Autodesk Inventor part; units mm, degrees
(part 3 of 6)
  line L1773 (-14.7808, 26.7541) -> (-14.5927, 26.602)
  line L1774 (-14.5927, 26.602) -> (-14.4184, 26.455)
  line L1775 (-14.4184, 26.455) -> (-14.2558, 26.312)
  line L1776 (-14.2558, 26.312) -> (-14.1046, 26.1732)
  line L1777 (-14.1046, 26.1732) -> (-13.9666, 26.0412)
  line L1778 (-13.9666, 26.0412) -> (-13.8398, 25.9146)
  line L1779 (-13.8398, 25.9146) -> (-13.5974, 25.6603)
  line L1780 (-13.5974, 25.6603) -> (-13.5605, 25.6314)
  line L1781 (-13.5605, 25.6314) -> (-13.5287, 25.6153)
  line L1782 (-13.5287, 25.6153) -> (-13.5023, 25.6116)
  line L1783 (-13.5023, 25.6116) -> (-13.4865, 25.6168)
  line L1784 (-13.4865, 25.6168) -> (-13.143, 25.7946)
  line L1785 (-13.143, 25.7946) -> (-12.7973, 25.968)
  line L1786 (-12.7973, 25.968) -> (-12.7837, 25.9777)
  line L1787 (-12.7837, 25.9777) -> (-12.7712, 26.0012)
  line L1788 (-12.7712, 26.0012) -> (-12.7656, 26.0365)
  line L1789 (-12.7656, 26.0365) -> (-12.7672, 26.0833)
  line L1790 (-12.7672, 26.0833) -> (-12.8305, 26.4288)
  line L1791 (-12.8305, 26.4288) -> (-12.8584, 26.6059)
  line L1792 (-12.8584, 26.6059) -> (-12.8841, 26.7951)
  line L1793 (-12.8841, 26.7951) -> (-12.9075, 26.9989)
  line L1794 (-12.9075, 26.9989) -> (-12.9276, 27.2145)
  line L1795 (-12.9276, 27.2145) -> (-12.9441, 27.442)
  line L1796 (-12.9441, 27.442) -> (-12.9565, 27.6836)
  line L1797 (-12.9565, 27.6836) -> (-12.9642, 27.9367)
  line L1798 (-12.9642, 27.9367) -> (-12.9667, 28.1579)
  arc A57 (-12.249, 28.4774) -> (-12.9667, 28.1579) centre (0, 0) ccw
  line L1799 (-12.249, 28.4774) -> (-12.0862, 28.3276)
  line L1800 (-12.0862, 28.3276) -> (-11.9033, 28.1525)
  line L1801 (-11.9033, 28.1525) -> (-11.7321, 27.9817)
  line L1802 (-11.7321, 27.9817) -> (-11.5741, 27.8172)
  line L1803 (-11.5741, 27.8172) -> (-11.4273, 27.6579)
  line L1804 (-11.4273, 27.6579) -> (-11.2915, 27.5042)
  line L1805 (-11.2915, 27.5042) -> (-11.1681, 27.3584)
  line L1806 (-11.1681, 27.3584) -> (-11.0551, 27.2193)
  line L1807 (-11.0551, 27.2193) -> (-10.8407, 26.941)
  line L1808 (-10.8407, 26.941) -> (-10.807, 26.9085)
  line L1809 (-10.807, 26.9085) -> (-10.777, 26.8891)
  line L1810 (-10.777, 26.8891) -> (-10.7512, 26.8826)
  line L1811 (-10.7512, 26.8826) -> (-10.7349, 26.8862)
  line L1812 (-10.7349, 26.8862) -> (-10.3748, 27.0272)
  line L1813 (-10.3748, 27.0272) -> (-10.0128, 27.1634)
  line L1814 (-10.0128, 27.1634) -> (-9.9983, 27.1717)
  line L1815 (-9.9983, 27.1717) -> (-9.9834, 27.1937)
  line L1816 (-9.9834, 27.1937) -> (-9.9741, 27.2282)
  line L1817 (-9.9741, 27.2282) -> (-9.9708, 27.2749)
  line L1818 (-9.9708, 27.2749) -> (-9.9977, 27.6252)
  line L1819 (-9.9977, 27.6252) -> (-10.0069, 27.8042)
  line L1820 (-10.0069, 27.8042) -> (-10.0127, 27.995)
  line L1821 (-10.0127, 27.995) -> (-10.0146, 28.2002)
  line L1822 (-10.0146, 28.2002) -> (-10.0121, 28.4168)
  line L1823 (-10.0121, 28.4168) -> (-10.0047, 28.6447)
  line L1824 (-10.0047, 28.6447) -> (-9.9918, 28.8863)
  line L1825 (-9.9918, 28.8863) -> (-9.973, 29.1388)
  line L1826 (-9.973, 29.1388) -> (-9.9523, 29.359)
  arc A58 (-9.2052, 29.6018) -> (-9.9523, 29.359) centre (0, 0) ccw
  line L1827 (-9.2052, 29.6018) -> (-9.059, 29.4358)
  line L1828 (-9.059, 29.4358) -> (-8.8954, 29.2425)
  line L1829 (-8.8954, 29.2425) -> (-8.7429, 29.0547)
  line L1830 (-8.7429, 29.0547) -> (-8.603, 28.8746)
  line L1831 (-8.603, 28.8746) -> (-8.4737, 28.7009)
  line L1832 (-8.4737, 28.7009) -> (-8.3547, 28.5338)
  line L1833 (-8.3547, 28.5338) -> (-8.2472, 28.3759)
  line L1834 (-8.2472, 28.3759) -> (-8.1494, 28.2257)
  line L1835 (-8.1494, 28.2257) -> (-7.9652, 27.9266)
  line L1836 (-7.9652, 27.9266) -> (-7.9351, 27.8907)
  line L1837 (-7.9351, 27.8907) -> (-7.9073, 27.8683)
  line L1838 (-7.9073, 27.8683) -> (-7.8823, 27.8592)
  line L1839 (-7.8823, 27.8592) -> (-7.8657, 27.861)
  line L1840 (-7.8657, 27.861) -> (-7.4928, 27.9636)
  line L1841 (-7.4928, 27.9636) -> (-7.1186, 28.0612)
  line L1842 (-7.1186, 28.0612) -> (-7.1033, 28.0679)
  line L1843 (-7.1033, 28.0679) -> (-7.0862, 28.0883)
  line L1844 (-7.0862, 28.0883) -> (-7.0733, 28.1216)
  line L1845 (-7.0733, 28.1216) -> (-7.0652, 28.1677)
  line L1846 (-7.0652, 28.1677) -> (-7.0553, 28.5189)
  line L1847 (-7.0553, 28.5189) -> (-7.0457, 28.6979)
  line L1848 (-7.0457, 28.6979) -> (-7.0315, 28.8883)
  line L1849 (-7.0315, 28.8883) -> (-7.012, 29.0926)
  line L1850 (-7.012, 29.0926) -> (-6.9869, 29.3077)
  line L1851 (-6.9869, 29.3077) -> (-6.9557, 29.5336)
  line L1852 (-6.9557, 29.5336) -> (-6.9177, 29.7725)
  line L1853 (-6.9177, 29.7725) -> (-6.8726, 30.0216)
  line L1854 (-6.8726, 30.0216) -> (-6.829, 30.2385)
  arc A59 (-6.0605, 30.4018) -> (-6.829, 30.2385) centre (0, 0) ccw
  line L1855 (-6.0605, 30.4018) -> (-5.9325, 30.2214)
  line L1856 (-5.9325, 30.2214) -> (-5.79, 30.0122)
  line L1857 (-5.79, 30.0122) -> (-5.658, 29.8094)
  line L1858 (-5.658, 29.8094) -> (-5.5376, 29.6157)
  line L1859 (-5.5376, 29.6157) -> (-5.4272, 29.4294)
  line L1860 (-5.4272, 29.4294) -> (-5.3263, 29.2508)
  line L1861 (-5.3263, 29.2508) -> (-5.2359, 29.0826)
  line L1862 (-5.2359, 29.0826) -> (-5.1544, 28.9229)
  line L1863 (-5.1544, 28.9229) -> (-5.0025, 28.6062)
  line L1864 (-5.0025, 28.6062) -> (-4.9763, 28.5674)
  line L1865 (-4.9763, 28.5674) -> (-4.951, 28.5421)
  line L1866 (-4.951, 28.5421) -> (-4.927, 28.5305)
  line L1867 (-4.927, 28.5305) -> (-4.9104, 28.5306)
  line L1868 (-4.9104, 28.5306) -> (-4.5288, 28.5936)
  line L1869 (-4.5288, 28.5936) -> (-4.1464, 28.6516)
  line L1870 (-4.1464, 28.6516) -> (-4.1305, 28.6567)
  line L1871 (-4.1305, 28.6567) -> (-4.1114, 28.6751)
  line L1872 (-4.1114, 28.6751) -> (-4.0951, 28.7069)
  line L1873 (-4.0951, 28.7069) -> (-4.0822, 28.7519)
  line L1874 (-4.0822, 28.7519) -> (-4.0356, 29.1001)
  line L1875 (-4.0356, 29.1001) -> (-4.0074, 29.2771)
  line L1876 (-4.0074, 29.2771) -> (-3.9734, 29.465)
  line L1877 (-3.9734, 29.465) -> (-3.9326, 29.6661)
  line L1878 (-3.9326, 29.6661) -> (-3.8852, 29.8774)
  line L1879 (-3.8852, 29.8774) -> (-3.8305, 30.0989)
  line L1880 (-3.8305, 30.0989) -> (-3.7677, 30.3325)
  line L1881 (-3.7677, 30.3325) -> (-3.6968, 30.5755)
  line L1882 (-3.6968, 30.5755) -> (-3.6308, 30.7866)
  arc A60 (-2.8495, 30.8688) -> (-3.6308, 30.7866) centre (0, 0) ccw
  line L1883 (-2.8495, 30.8688) -> (-2.741, 30.676)
  line L1884 (-2.741, 30.676) -> (-2.6211, 30.453)
  line L1885 (-2.6211, 30.453) -> (-2.5111, 30.2376)
  line L1886 (-2.5111, 30.2376) -> (-2.4116, 30.0323)
  line L1887 (-2.4116, 30.0323) -> (-2.3213, 29.8355)
  line L1888 (-2.3213, 29.8355) -> (-2.2396, 29.6473)
  line L1889 (-2.2396, 29.6473) -> (-2.1673, 29.4705)
  line L1890 (-2.1673, 29.4705) -> (-2.1029, 29.3033)
  line L1891 (-2.1029, 29.3033) -> (-1.9849, 28.9724)
  line L1892 (-1.9849, 28.9724) -> (-1.9629, 28.931)
  line L1893 (-1.9629, 28.931) -> (-1.9404, 28.9033)
  line L1894 (-1.9404, 28.9033) -> (-1.9178, 28.8892)
  line L1895 (-1.9178, 28.8892) -> (-1.9012, 28.8876)
  line L1896 (-1.9012, 28.8876) -> (-1.5151, 28.9103)
  line L1897 (-1.5151, 28.9103) -> (-1.1288, 28.9281)
  line L1898 (-1.1288, 28.9281) -> (-1.1124, 28.9314)
  line L1899 (-1.1124, 28.9314) -> (-1.0915, 28.9478)
  line L1900 (-1.0915, 28.9478) -> (-1.0719, 28.9777)
  line L1901 (-1.0719, 28.9777) -> (-1.0544, 29.0211)
  line L1902 (-1.0544, 29.0211) -> (-0.9717, 29.3626)
  line L1903 (-0.9717, 29.3626) -> (-0.9251, 29.5356)
  line L1904 (-0.9251, 29.5356) -> (-0.8717, 29.719)
  line L1905 (-0.8717, 29.719) -> (-0.8101, 29.9147)
  line L1906 (-0.8101, 29.9147) -> (-0.7408, 30.1199)
  line L1907 (-0.7408, 30.1199) -> (-0.6634, 30.3344)
  line L1908 (-0.6634, 30.3344) -> (-0.5765, 30.5601)
  line L1909 (-0.5765, 30.5601) -> (-0.4805, 30.7945)
  line L1910 (-0.4805, 30.7945) -> (-0.3928, 30.9975)
  arc A61 (0.3928, 30.9975) -> (-0.3928, 30.9975) centre (0, 0) ccw
  line L1911 (0.3928, 30.9975) -> (0.4805, 30.7945)
  line L1912 (0.4805, 30.7945) -> (0.5765, 30.5601)
  line L1913 (0.5765, 30.5601) -> (0.6634, 30.3344)
  line L1914 (0.6634, 30.3344) -> (0.7408, 30.1199)
  line L1915 (0.7408, 30.1199) -> (0.8101, 29.9147)
  line L1916 (0.8101, 29.9147) -> (0.8717, 29.719)
  line L1917 (0.8717, 29.719) -> (0.9251, 29.5356)
  line L1918 (0.9251, 29.5356) -> (0.9717, 29.3626)
  line L1919 (0.9717, 29.3626) -> (1.0544, 29.0211)
  line L1920 (1.0544, 29.0211) -> (1.0719, 28.9777)
  line L1921 (1.0719, 28.9777) -> (1.0915, 28.9478)
  line L1922 (1.0915, 28.9478) -> (1.1124, 28.9314)
  line L1923 (1.1124, 28.9314) -> (1.1288, 28.9281)
  line L1924 (1.1288, 28.9281) -> (1.5151, 28.9103)
  line L1925 (1.5151, 28.9103) -> (1.9012, 28.8876)
  line L1926 (1.9012, 28.8876) -> (1.9178, 28.8892)
  line L1927 (1.9178, 28.8892) -> (1.9404, 28.9033)
  line L1928 (1.9404, 28.9033) -> (1.9629, 28.931)
  line L1929 (1.9629, 28.931) -> (1.9849, 28.9724)
  line L1930 (1.9849, 28.9724) -> (2.1029, 29.3033)
  line L1931 (2.1029, 29.3033) -> (2.1673, 29.4705)
  line L1932 (2.1673, 29.4705) -> (2.2396, 29.6473)
  line L1933 (2.2396, 29.6473) -> (2.3213, 29.8355)
  line L1934 (2.3213, 29.8355) -> (2.4116, 30.0323)
  line L1935 (2.4116, 30.0323) -> (2.5111, 30.2376)
  line L1936 (2.5111, 30.2376) -> (2.6211, 30.453)
  line L1937 (2.6211, 30.453) -> (2.741, 30.676)
  line L1938 (2.741, 30.676) -> (2.8495, 30.8688)
  arc A62 (3.6308, 30.7866) -> (2.8495, 30.8688) centre (0, 0) ccw
  line L1939 (3.6308, 30.7866) -> (3.6968, 30.5755)
  line L1940 (3.6968, 30.5755) -> (3.7677, 30.3325)
  line L1941 (3.7677, 30.3325) -> (3.8305, 30.0989)
  line L1942 (3.8305, 30.0989) -> (3.8852, 29.8774)
  line L1943 (3.8852, 29.8774) -> (3.9326, 29.6661)
  line L1944 (3.9326, 29.6661) -> (3.9734, 29.465)
  line L1945 (3.9734, 29.465) -> (4.0074, 29.2771)
  line L1946 (4.0074, 29.2771) -> (4.0356, 29.1001)
  line L1947 (4.0356, 29.1001) -> (4.0822, 28.7519)
  line L1948 (4.0822, 28.7519) -> (4.0951, 28.7069)
  line L1949 (4.0951, 28.7069) -> (4.1114, 28.6751)
  line L1950 (4.1114, 28.6751) -> (4.1305, 28.6567)
  line L1951 (4.1305, 28.6567) -> (4.1464, 28.6516)
  line L1952 (4.1464, 28.6516) -> (4.5288, 28.5936)
  line L1953 (4.5288, 28.5936) -> (4.9104, 28.5306)
  line L1954 (4.9104, 28.5306) -> (4.927, 28.5305)
  line L1955 (4.927, 28.5305) -> (4.951, 28.5421)
  line L1956 (4.951, 28.5421) -> (4.9763, 28.5674)
  line L1957 (4.9763, 28.5674) -> (5.0025, 28.6062)
  line L1958 (5.0025, 28.6062) -> (5.1544, 28.9229)
  line L1959 (5.1544, 28.9229) -> (5.2359, 29.0826)
  line L1960 (5.2359, 29.0826) -> (5.3263, 29.2508)
  line L1961 (5.3263, 29.2508) -> (5.4272, 29.4294)
  line L1962 (5.4272, 29.4294) -> (5.5376, 29.6157)
  line L1963 (5.5376, 29.6157) -> (5.658, 29.8094)
  line L1964 (5.658, 29.8094) -> (5.79, 30.0122)
  line L1965 (5.79, 30.0122) -> (5.9325, 30.2214)
  line L1966 (5.9325, 30.2214) -> (6.0605, 30.4018)
  arc A63 (6.829, 30.2385) -> (6.0605, 30.4018) centre (0, 0) ccw
  line L1967 (6.829, 30.2385) -> (6.8726, 30.0216)
  line L1968 (6.8726, 30.0216) -> (6.9177, 29.7725)
  line L1969 (6.9177, 29.7725) -> (6.9557, 29.5336)
  line L1970 (6.9557, 29.5336) -> (6.9869, 29.3077)
  line L1971 (6.9869, 29.3077) -> (7.012, 29.0926)
  line L1972 (7.012, 29.0926) -> (7.0315, 28.8883)
  line L1973 (7.0315, 28.8883) -> (7.0457, 28.6979)
  line L1974 (7.0457, 28.6979) -> (7.0553, 28.5189)
  line L1975 (7.0553, 28.5189) -> (7.0652, 28.1677)
  line L1976 (7.0652, 28.1677) -> (7.0733, 28.1216)
  line L1977 (7.0733, 28.1216) -> (7.0862, 28.0883)
  line L1978 (7.0862, 28.0883) -> (7.1033, 28.0679)
  line L1979 (7.1033, 28.0679) -> (7.1186, 28.0612)
  line L1980 (7.1186, 28.0612) -> (7.4928, 27.9636)
  line L1981 (7.4928, 27.9636) -> (7.8657, 27.861)
  line L1982 (7.8657, 27.861) -> (7.8823, 27.8592)
  line L1983 (7.8823, 27.8592) -> (7.9073, 27.8683)
  line L1984 (7.9073, 27.8683) -> (7.9351, 27.8907)
  line L1985 (7.9351, 27.8907) -> (7.9652, 27.9266)
  line L1986 (7.9652, 27.9266) -> (8.1494, 28.2257)
  line L1987 (8.1494, 28.2257) -> (8.2472, 28.3759)
  line L1988 (8.2472, 28.3759) -> (8.3547, 28.5338)
  line L1989 (8.3547, 28.5338) -> (8.4737, 28.7009)
  line L1990 (8.4737, 28.7009) -> (8.603, 28.8746)
  line L1991 (8.603, 28.8746) -> (8.7429, 29.0547)
  line L1992 (8.7429, 29.0547) -> (8.8954, 29.2425)
  line L1993 (8.8954, 29.2425) -> (9.059, 29.4358)
  line L1994 (9.059, 29.4358) -> (9.2052, 29.6018)
  arc A64 (9.9523, 29.359) -> (9.2052, 29.6018) centre (0, 0) ccw
  line L1995 (9.9523, 29.359) -> (9.973, 29.1388)
  line L1996 (9.973, 29.1388) -> (9.9918, 28.8863)
  line L1997 (9.9918, 28.8863) -> (10.0047, 28.6447)
  line L1998 (10.0047, 28.6447) -> (10.0121, 28.4168)
  line L1999 (10.0121, 28.4168) -> (10.0146, 28.2002)
  line L2000 (10.0146, 28.2002) -> (10.0127, 27.995)
  line L2001 (10.0127, 27.995) -> (10.0069, 27.8042)
  line L2002 (10.0069, 27.8042) -> (9.9977, 27.6252)
  line L2003 (9.9977, 27.6252) -> (9.9708, 27.2749)
  line L2004 (9.9708, 27.2749) -> (9.9741, 27.2282)
  line L2005 (9.9741, 27.2282) -> (9.9834, 27.1937)
  line L2006 (9.9834, 27.1937) -> (9.9983, 27.1717)
  line L2007 (9.9983, 27.1717) -> (10.0128, 27.1634)
  line L2008 (10.0128, 27.1634) -> (10.3748, 27.0272)
  line L2009 (10.3748, 27.0272) -> (10.7349, 26.8862)
  line L2010 (10.7349, 26.8862) -> (10.7512, 26.8826)
  line L2011 (10.7512, 26.8826) -> (10.777, 26.8891)
  line L2012 (10.777, 26.8891) -> (10.807, 26.9085)
  line L2013 (10.807, 26.9085) -> (10.8407, 26.941)
  line L2014 (10.8407, 26.941) -> (11.0551, 27.2193)
  line L2015 (11.0551, 27.2193) -> (11.1681, 27.3584)
  line L2016 (11.1681, 27.3584) -> (11.2915, 27.5042)
  line L2017 (11.2915, 27.5042) -> (11.4273, 27.6579)
  line L2018 (11.4273, 27.6579) -> (11.5741, 27.8172)
  line L2019 (11.5741, 27.8172) -> (11.7321, 27.9817)
  line L2020 (11.7321, 27.9817) -> (11.9033, 28.1525)
  line L2021 (11.9033, 28.1525) -> (12.0862, 28.3276)
  line L2022 (12.0862, 28.3276) -> (12.249, 28.4774)
  arc A65 (12.9667, 28.1579) -> (12.249, 28.4774) centre (0, 0) ccw
  line L2023 (12.9667, 28.1579) -> (12.9642, 27.9367)
  line L2024 (12.9642, 27.9367) -> (12.9565, 27.6836)
  line L2025 (12.9565, 27.6836) -> (12.9441, 27.442)
  line L2026 (12.9441, 27.442) -> (12.9276, 27.2145)
  line L2027 (12.9276, 27.2145) -> (12.9075, 26.9989)
  line L2028 (12.9075, 26.9989) -> (12.8841, 26.7951)
  line L2029 (12.8841, 26.7951) -> (12.8584, 26.6059)
  line L2030 (12.8584, 26.6059) -> (12.8305, 26.4288)
  line L2031 (12.8305, 26.4288) -> (12.7672, 26.0833)
  line L2032 (12.7672, 26.0833) -> (12.7656, 26.0365)
  line L2033 (12.7656, 26.0365) -> (12.7712, 26.0012)
  line L2034 (12.7712, 26.0012) -> (12.7837, 25.9777)
  line L2035 (12.7837, 25.9777) -> (12.7973, 25.968)
  line L2036 (12.7973, 25.968) -> (13.143, 25.7946)
  line L2037 (13.143, 25.7946) -> (13.4865, 25.6168)
  line L2038 (13.4865, 25.6168) -> (13.5023, 25.6116)
  line L2039 (13.5023, 25.6116) -> (13.5287, 25.6153)
  line L2040 (13.5287, 25.6153) -> (13.5605, 25.6314)
  line L2041 (13.5605, 25.6314) -> (13.5974, 25.6603)
  line L2042 (13.5974, 25.6603) -> (13.8398, 25.9146)
  line L2043 (13.8398, 25.9146) -> (13.9666, 26.0412)
  line L2044 (13.9666, 26.0412) -> (14.1046, 26.1732)
  line L2045 (14.1046, 26.1732) -> (14.2558, 26.312)
  line L2046 (14.2558, 26.312) -> (14.4184, 26.455)
  line L2047 (14.4184, 26.455) -> (14.5927, 26.602)
  line L2048 (14.5927, 26.602) -> (14.7808, 26.7541)
  line L2049 (14.7808, 26.7541) -> (14.9811, 26.9091)
  line L2050 (14.9811, 26.9091) -> (15.1586, 27.041)
  arc A66 (15.8389, 26.6482) -> (15.1586, 27.041) centre (0, 0) ccw
  line L2051 (15.8389, 26.6482) -> (15.8134, 26.4285)
  line L2052 (15.8134, 26.4285) -> (15.7793, 26.1776)
  line L2053 (15.7793, 26.1776) -> (15.7417, 25.9387)
  line L2054 (15.7417, 25.9387) -> (15.7015, 25.7142)
  line L2055 (15.7015, 25.7142) -> (15.6589, 25.5018)
  line L2056 (15.6589, 25.5018) -> (15.6144, 25.3015)
  line L2057 (15.6144, 25.3015) -> (15.569, 25.1161)
  line L2058 (15.569, 25.1161) -> (15.5228, 24.9429)
  line L2059 (15.5228, 24.9429) -> (15.4237, 24.6058)
  line L2060 (15.4237, 24.6058) -> (15.4172, 24.5595)
  line L2061 (15.4172, 24.5595) -> (15.4191, 24.5238)
  line L2062 (15.4191, 24.5238) -> (15.4291, 24.4991)
  line L2063 (15.4291, 24.4991) -> (15.4416, 24.488)
  line L2064 (15.4416, 24.488) -> (15.7673, 24.2795)
  line L2065 (15.7673, 24.2795) -> (16.0903, 24.0668)
  line L2066 (16.0903, 24.0668) -> (16.1055, 24.0599)
  line L2067 (16.1055, 24.0599) -> (16.1321, 24.0608)
  line L2068 (16.1321, 24.0608) -> (16.1655, 24.0735)
  line L2069 (16.1655, 24.0735) -> (16.2052, 24.0984)
  line L2070 (16.2052, 24.0984) -> (16.4728, 24.326)
  line L2071 (16.4728, 24.326) -> (16.6122, 24.4386)
  line L2072 (16.6122, 24.4386) -> (16.7632, 24.5555)
  line L2073 (16.7632, 24.5555) -> (16.928, 24.6777)
  line L2074 (16.928, 24.6777) -> (17.1047, 24.8029)
  line L2075 (17.1047, 24.8029) -> (17.2934, 24.931)
  line L2076 (17.2934, 24.931) -> (17.4964, 25.0625)
  line L2077 (17.4964, 25.0625) -> (17.7118, 25.1957)
  line L2078 (17.7118, 25.1957) -> (17.9021, 25.3084)
  arc A67 (18.5377, 24.8466) -> (17.9021, 25.3084) centre (0, 0) ccw
  line L2079 (18.5377, 24.8466) -> (18.4893, 24.6308)
  line L2080 (18.4893, 24.6308) -> (18.4292, 24.3848)
  line L2081 (18.4292, 24.3848) -> (18.3668, 24.1511)
  line L2082 (18.3668, 24.1511) -> (18.3034, 23.932)
  line L2083 (18.3034, 23.932) -> (18.2388, 23.7253)
  line L2084 (18.2388, 23.7253) -> (18.1736, 23.5308)
  line L2085 (18.1736, 23.5308) -> (18.1091, 23.3511)
  line L2086 (18.1091, 23.3511) -> (18.045, 23.1837)
  line L2087 (18.045, 23.1837) -> (17.9112, 22.8588)
  line L2088 (17.9112, 22.8588) -> (17.8999, 22.8134)
  line L2089 (17.8999, 22.8134) -> (17.8981, 22.7777)
  line L2090 (17.8981, 22.7777) -> (17.9055, 22.7521)
  line L2091 (17.9055, 22.7521) -> (17.9167, 22.7398)
  line L2092 (17.9167, 22.7398) -> (18.2188, 22.4984)
  line L2093 (18.2188, 22.4984) -> (18.5178, 22.2531)
  line L2094 (18.5178, 22.2531) -> (18.5322, 22.2446)
  line L2095 (18.5322, 22.2446) -> (18.5587, 22.2427)
  line L2096 (18.5587, 22.2427) -> (18.5933, 22.2519)
  line L2097 (18.5933, 22.2519) -> (18.6353, 22.2724)
  line L2098 (18.6353, 22.2724) -> (18.9253, 22.4708)
  line L2099 (18.9253, 22.4708) -> (19.0757, 22.5683)
  line L2100 (19.0757, 22.5683) -> (19.2381, 22.6688)
  line L2101 (19.2381, 22.6688) -> (19.4148, 22.773)
  line L2102 (19.4148, 22.773) -> (19.6036, 22.8791)
  line L2103 (19.6036, 22.8791) -> (19.8047, 22.9867)
  line L2104 (19.8047, 22.9867) -> (20.0203, 23.0963)
  line L2105 (20.0203, 23.0963) -> (20.2484, 23.2063)
  line L2106 (20.2484, 23.2063) -> (20.4495, 23.2985)
  arc A68 (21.0333, 22.7728) -> (20.4495, 23.2985) centre (0, 0) ccw
  line L2107 (21.0333, 22.7728) -> (20.9626, 22.5632)
  line L2108 (20.9626, 22.5632) -> (20.8771, 22.3249)
  line L2109 (20.8771, 22.3249) -> (20.7906, 22.099)
  line L2110 (20.7906, 22.099) -> (20.7047, 21.8877)
  line L2111 (20.7047, 21.8877) -> (20.6189, 21.6889)
  line L2112 (20.6189, 21.6889) -> (20.5336, 21.5022)
  line L2113 (20.5336, 21.5022) -> (20.4507, 21.3302)
  line L2114 (20.4507, 21.3302) -> (20.3695, 21.1705)
  line L2115 (20.3695, 21.1705) -> (20.2025, 20.8614)
  line L2116 (20.2025, 20.8614) -> (20.1865, 20.8174)
  line L2117 (20.1865, 20.8174) -> (20.181, 20.7821)
  line L2118 (20.181, 20.7821) -> (20.1856, 20.7559)
  line L2119 (20.1856, 20.7559) -> (20.1955, 20.7424)
  line L2120 (20.1955, 20.7424) -> (20.4707, 20.4707)
  line L2121 (20.4707, 20.4707) -> (20.7424, 20.1955)
  line L2122 (20.7424, 20.1955) -> (20.7559, 20.1856)
  line L2123 (20.7559, 20.1856) -> (20.7821, 20.181)
  line L2124 (20.7821, 20.181) -> (20.8174, 20.1865)
  line L2125 (20.8174, 20.1865) -> (20.8614, 20.2025)
  line L2126 (20.8614, 20.2025) -> (21.1705, 20.3695)
  line L2127 (21.1705, 20.3695) -> (21.3302, 20.4507)
  line L2128 (21.3302, 20.4507) -> (21.5022, 20.5336)
  line L2129 (21.5022, 20.5336) -> (21.6889, 20.6189)
  line L2130 (21.6889, 20.6189) -> (21.8877, 20.7047)
  line L2131 (21.8877, 20.7047) -> (22.099, 20.7906)
  line L2132 (22.099, 20.7906) -> (22.3249, 20.8771)
  line L2133 (22.3249, 20.8771) -> (22.5632, 20.9626)
  line L2134 (22.5632, 20.9626) -> (22.7728, 21.0333)
  arc A69 (23.2985, 20.4495) -> (22.7728, 21.0333) centre (0, 0) ccw
  line L2135 (23.2985, 20.4495) -> (23.2063, 20.2484)
  line L2136 (23.2063, 20.2484) -> (23.0963, 20.0203)
  line L2137 (23.0963, 20.0203) -> (22.9867, 19.8047)
  line L2138 (22.9867, 19.8047) -> (22.8791, 19.6036)
  line L2139 (22.8791, 19.6036) -> (22.773, 19.4148)
  line L2140 (22.773, 19.4148) -> (22.6688, 19.2381)
  line L2141 (22.6688, 19.2381) -> (22.5683, 19.0757)
  line L2142 (22.5683, 19.0757) -> (22.4708, 18.9253)
  line L2143 (22.4708, 18.9253) -> (22.2724, 18.6353)
  line L2144 (22.2724, 18.6353) -> (22.2519, 18.5933)
  line L2145 (22.2519, 18.5933) -> (22.2427, 18.5587)
  line L2146 (22.2427, 18.5587) -> (22.2446, 18.5322)
  line L2147 (22.2446, 18.5322) -> (22.2531, 18.5178)
  line L2148 (22.2531, 18.5178) -> (22.4984, 18.2188)
  line L2149 (22.4984, 18.2188) -> (22.7398, 17.9167)
  line L2150 (22.7398, 17.9167) -> (22.7521, 17.9055)
  line L2151 (22.7521, 17.9055) -> (22.7777, 17.8981)
  line L2152 (22.7777, 17.8981) -> (22.8134, 17.8999)
  line L2153 (22.8134, 17.8999) -> (22.8588, 17.9112)
  line L2154 (22.8588, 17.9112) -> (23.1837, 18.045)
  line L2155 (23.1837, 18.045) -> (23.3511, 18.1091)
  line L2156 (23.3511, 18.1091) -> (23.5308, 18.1736)
  line L2157 (23.5308, 18.1736) -> (23.7253, 18.2388)
  line L2158 (23.7253, 18.2388) -> (23.932, 18.3034)
  line L2159 (23.932, 18.3034) -> (24.1511, 18.3668)
  line L2160 (24.1511, 18.3668) -> (24.3848, 18.4292)
  line L2161 (24.3848, 18.4292) -> (24.6308, 18.4893)
  line L2162 (24.6308, 18.4893) -> (24.8466, 18.5377)
  arc A70 (25.3084, 17.9021) -> (24.8466, 18.5377) centre (0, 0) ccw
  line L2163 (25.3084, 17.9021) -> (25.1957, 17.7118)
  line L2164 (25.1957, 17.7118) -> (25.0625, 17.4964)
  line L2165 (25.0625, 17.4964) -> (24.931, 17.2934)
  line L2166 (24.931, 17.2934) -> (24.8029, 17.1047)
  line L2167 (24.8029, 17.1047) -> (24.6777, 16.928)
  line L2168 (24.6777, 16.928) -> (24.5555, 16.7632)
  line L2169 (24.5555, 16.7632) -> (24.4386, 16.6122)
  line L2170 (24.4386, 16.6122) -> (24.326, 16.4728)
  line L2171 (24.326, 16.4728) -> (24.0984, 16.2052)
  line L2172 (24.0984, 16.2052) -> (24.0735, 16.1655)
  line L2173 (24.0735, 16.1655) -> (24.0608, 16.1321)
  line L2174 (24.0608, 16.1321) -> (24.0599, 16.1055)
  line L2175 (24.0599, 16.1055) -> (24.0668, 16.0903)
  line L2176 (24.0668, 16.0903) -> (24.2795, 15.7673)
  line L2177 (24.2795, 15.7673) -> (24.488, 15.4416)
  line L2178 (24.488, 15.4416) -> (24.4991, 15.4291)
  line L2179 (24.4991, 15.4291) -> (24.5238, 15.4191)
  line L2180 (24.5238, 15.4191) -> (24.5595, 15.4172)
  line L2181 (24.5595, 15.4172) -> (24.6058, 15.4237)
  line L2182 (24.6058, 15.4237) -> (24.9429, 15.5228)
  line L2183 (24.9429, 15.5228) -> (25.1161, 15.569)
  line L2184 (25.1161, 15.569) -> (25.3015, 15.6144)
  line L2185 (25.3015, 15.6144) -> (25.5018, 15.6589)
  line L2186 (25.5018, 15.6589) -> (25.7142, 15.7015)
  line L2187 (25.7142, 15.7015) -> (25.9387, 15.7417)
  line L2188 (25.9387, 15.7417) -> (26.1776, 15.7793)
  line L2189 (26.1776, 15.7793) -> (26.4285, 15.8134)
  line L2190 (26.4285, 15.8134) -> (26.6482, 15.8389)
  arc A71 (27.041, 15.1586) -> (26.6482, 15.8389) centre (0, 0) ccw
  line L2191 (27.041, 15.1586) -> (26.9091, 14.9811)
  line L2192 (26.9091, 14.9811) -> (26.7541, 14.7808)
  line L2193 (26.7541, 14.7808) -> (26.602, 14.5927)
  line L2194 (26.602, 14.5927) -> (26.455, 14.4184)
  line L2195 (26.455, 14.4184) -> (26.312, 14.2558)
  line L2196 (26.312, 14.2558) -> (26.1732, 14.1046)
  line L2197 (26.1732, 14.1046) -> (26.0412, 13.9666)
  line L2198 (26.0412, 13.9666) -> (25.9146, 13.8398)
  line L2199 (25.9146, 13.8398) -> (25.6603, 13.5974)
  line L2200 (25.6603, 13.5974) -> (25.6314, 13.5605)
  line L2201 (25.6314, 13.5605) -> (25.6153, 13.5287)
  line L2202 (25.6153, 13.5287) -> (25.6116, 13.5023)
  line L2203 (25.6116, 13.5023) -> (25.6168, 13.4865)
  line L2204 (25.6168, 13.4865) -> (25.7946, 13.143)
  line L2205 (25.7946, 13.143) -> (25.968, 12.7973)
  line L2206 (25.968, 12.7973) -> (25.9777, 12.7837)
  line L2207 (25.9777, 12.7837) -> (26.0012, 12.7712)
  line L2208 (26.0012, 12.7712) -> (26.0365, 12.7656)
  line L2209 (26.0365, 12.7656) -> (26.0833, 12.7672)
  line L2210 (26.0833, 12.7672) -> (26.4288, 12.8305)
  line L2211 (26.4288, 12.8305) -> (26.6059, 12.8584)
  line L2212 (26.6059, 12.8584) -> (26.7951, 12.8841)
  line L2213 (26.7951, 12.8841) -> (26.9989, 12.9075)
  line L2214 (26.9989, 12.9075) -> (27.2145, 12.9276)
  line L2215 (27.2145, 12.9276) -> (27.442, 12.9441)
  line L2216 (27.442, 12.9441) -> (27.6836, 12.9565)
  line L2217 (27.6836, 12.9565) -> (27.9367, 12.9642)
  line L2218 (27.9367, 12.9642) -> (28.1579, 12.9667)
  arc A72 (28.4774, 12.249) -> (28.1579, 12.9667) centre (0, 0) ccw
  line L2219 (28.4774, 12.249) -> (28.3276, 12.0862)
  line L2220 (28.3276, 12.0862) -> (28.1525, 11.9033)
  line L2221 (28.1525, 11.9033) -> (27.9817, 11.7321)
  line L2222 (27.9817, 11.7321) -> (27.8172, 11.5741)
  line L2223 (27.8172, 11.5741) -> (27.6579, 11.4273)
  line L2224 (27.6579, 11.4273) -> (27.5042, 11.2915)
  line L2225 (27.5042, 11.2915) -> (27.3584, 11.1681)
  line L2226 (27.3584, 11.1681) -> (27.2193, 11.0551)
  line L2227 (27.2193, 11.0551) -> (26.941, 10.8407)
  line L2228 (26.941, 10.8407) -> (26.9085, 10.807)
  line L2229 (26.9085, 10.807) -> (26.8891, 10.777)
  line L2230 (26.8891, 10.777) -> (26.8826, 10.7512)
  line L2231 (26.8826, 10.7512) -> (26.8862, 10.7349)
  line L2232 (26.8862, 10.7349) -> (27.0272, 10.3748)
  line L2233 (27.0272, 10.3748) -> (27.1634, 10.0128)
  line L2234 (27.1634, 10.0128) -> (27.1717, 9.9983)
  line L2235 (27.1717, 9.9983) -> (27.1937, 9.9834)
  line L2236 (27.1937, 9.9834) -> (27.2282, 9.9741)
  line L2237 (27.2282, 9.9741) -> (27.2749, 9.9708)
  line L2238 (27.2749, 9.9708) -> (27.6252, 9.9977)
  line L2239 (27.6252, 9.9977) -> (27.8042, 10.0069)
  line L2240 (27.8042, 10.0069) -> (27.995, 10.0127)
  line L2241 (27.995, 10.0127) -> (28.2002, 10.0146)
  line L2242 (28.2002, 10.0146) -> (28.4168, 10.0121)
  line L2243 (28.4168, 10.0121) -> (28.6447, 10.0047)
  line L2244 (28.6447, 10.0047) -> (28.8863, 9.9918)
  line L2245 (28.8863, 9.9918) -> (29.1388, 9.973)
  line L2246 (29.1388, 9.973) -> (29.359, 9.9523)
  arc A73 (29.6018, 9.2052) -> (29.359, 9.9523) centre (0, 0) ccw
  line L2247 (29.6018, 9.2052) -> (29.4358, 9.059)
  line L2248 (29.4358, 9.059) -> (29.2425, 8.8954)
  line L2249 (29.2425, 8.8954) -> (29.0547, 8.7429)
  line L2250 (29.0547, 8.7429) -> (28.8746, 8.603)
  line L2251 (28.8746, 8.603) -> (28.7009, 8.4737)
  line L2252 (28.7009, 8.4737) -> (28.5338, 8.3547)
  line L2253 (28.5338, 8.3547) -> (28.3759, 8.2472)
  line L2254 (28.3759, 8.2472) -> (28.2257, 8.1494)
  line L2255 (28.2257, 8.1494) -> (27.9266, 7.9652)
  line L2256 (27.9266, 7.9652) -> (27.8907, 7.9351)
  line L2257 (27.8907, 7.9351) -> (27.8683, 7.9073)
  line L2258 (27.8683, 7.9073) -> (27.8592, 7.8823)
  line L2259 (27.8592, 7.8823) -> (27.861, 7.8657)
  line L2260 (27.861, 7.8657) -> (27.9636, 7.4928)
  line L2261 (27.9636, 7.4928) -> (28.0612, 7.1186)
  line L2262 (28.0612, 7.1186) -> (28.0679, 7.1033)
  line L2263 (28.0679, 7.1033) -> (28.0883, 7.0862)
  line L2264 (28.0883, 7.0862) -> (28.1216, 7.0733)
  line L2265 (28.1216, 7.0733) -> (28.1677, 7.0652)
  line L2266 (28.1677, 7.0652) -> (28.5189, 7.0553)
  line L2267 (28.5189, 7.0553) -> (28.6979, 7.0457)
  line L2268 (28.6979, 7.0457) -> (28.8883, 7.0315)
  line L2269 (28.8883, 7.0315) -> (29.0926, 7.012)
  line L2270 (29.0926, 7.012) -> (29.3077, 6.9869)
  line L2271 (29.3077, 6.9869) -> (29.5336, 6.9557)
  line L2272 (29.5336, 6.9557) -> (29.7725, 6.9177)
  line L2273 (29.7725, 6.9177) -> (30.0216, 6.8726)
  line L2274 (30.0216, 6.8726) -> (30.2385, 6.829)
  arc A74 (30.4018, 6.0605) -> (30.2385, 6.829) centre (0, 0) ccw
  line L2275 (30.4018, 6.0605) -> (30.2214, 5.9325)
  line L2276 (30.2214, 5.9325) -> (30.0122, 5.79)
  line L2277 (30.0122, 5.79) -> (29.8094, 5.658)
  line L2278 (29.8094, 5.658) -> (29.6157, 5.5376)
  line L2279 (29.6157, 5.5376) -> (29.4294, 5.4272)
  line L2280 (29.4294, 5.4272) -> (29.2508, 5.3263)
  line L2281 (29.2508, 5.3263) -> (29.0826, 5.2359)
  line L2282 (29.0826, 5.2359) -> (28.9229, 5.1544)
  line L2283 (28.9229, 5.1544) -> (28.6062, 5.0025)
  line L2284 (28.6062, 5.0025) -> (28.5674, 4.9763)
  line L2285 (28.5674, 4.9763) -> (28.5421, 4.951)
  line L2286 (28.5421, 4.951) -> (28.5305, 4.927)
  line L2287 (28.5305, 4.927) -> (28.5306, 4.9104)
  line L2288 (28.5306, 4.9104) -> (28.5936, 4.5288)
  line L2289 (28.5936, 4.5288) -> (28.6516, 4.1464)
  line L2290 (28.6516, 4.1464) -> (28.6567, 4.1305)
  line L2291 (28.6567, 4.1305) -> (28.6751, 4.1114)
  line L2292 (28.6751, 4.1114) -> (28.7069, 4.0951)
  line L2293 (28.7069, 4.0951) -> (28.7519, 4.0822)
  line L2294 (28.7519, 4.0822) -> (29.1001, 4.0356)
  line L2295 (29.1001, 4.0356) -> (29.2771, 4.0074)
  line L2296 (29.2771, 4.0074) -> (29.465, 3.9734)
  line L2297 (29.465, 3.9734) -> (29.6661, 3.9326)
  line L2298 (29.6661, 3.9326) -> (29.8774, 3.8852)
  line L2299 (29.8774, 3.8852) -> (30.0989, 3.8305)
  line L2300 (30.0989, 3.8305) -> (30.3325, 3.7677)
  line L2301 (30.3325, 3.7677) -> (30.5755, 3.6968)
  line L2302 (30.5755, 3.6968) -> (30.7866, 3.6308)
  arc A75 (30.8688, 2.8495) -> (30.7866, 3.6308) centre (0, 0) ccw
  line L2303 (30.8688, 2.8495) -> (30.676, 2.741)
  line L2304 (30.8694, -4.5708) -> (30.9098, -4.4161)
  line L2305 (30.9098, -4.4161) -> (30.9538, -4.2725)
  line L2306 (30.9538, -4.2725) -> (31.0003, -4.1408)
  line L2307 (31.0003, -4.1408) -> (31.0488, -4.0198)
  line L2308 (31.0488, -4.0198) -> (31.0977, -3.9112)
  line L2309 (31.0977, -3.9112) -> (31.1475, -3.8119)
  line L2310 (31.1475, -3.8119) -> (31.1956, -3.7252)
  line L2311 (31.1956, -3.7252) -> (31.2429, -3.6478)
  line L2312 (31.2429, -3.6478) -> (31.2875, -3.5813)
  line L2313 (31.2875, -3.5813) -> (31.3671, -3.477)
  line L2314 (31.3671, -3.477) -> (31.4285, -3.4089)
  line L2315 (31.4285, -3.4089) -> (31.466, -3.3746)
  line L2316 (31.466, -3.3746) -> (31.5668, -3.3141)
  line L2317 (31.5668, -3.3141) -> (31.6547, -3.2516)
  line L2318 (31.6547, -3.2516) -> (31.7296, -3.1879)
  line L2319 (31.7296, -3.1879) -> (31.7917, -3.1241)
  line L2320 (31.7917, -3.1241) -> (31.841, -3.0611)
  line L2321 (31.841, -3.0611) -> (31.8779, -2.9999)
  line L2322 (31.8779, -2.9999) -> (31.9025, -2.9414)
  line L2323 (31.9025, -2.9414) -> (31.9152, -2.8864)
  line L2324 (31.9152, -2.8864) -> (31.9163, -2.836)
  line L2325 (31.9163, -2.836) -> (31.9062, -2.7909)
  line L2326 (31.9062, -2.7909) -> (31.8916, -2.7611)
  line L2327 (31.8916, -2.7611) -> (31.8003, -2.6202)
  line L2328 (31.8003, -2.6202) -> (31.7132, -2.475)
  line L2329 (31.7132, -2.475) -> (31.631, -2.327)
  line L2330 (31.631, -2.327) -> (31.5546, -2.1774)
  line L2331 (31.5546, -2.1774) -> (31.5361, -2.1499)
  line L2332 (31.5361, -2.1499) -> (31.5021, -2.1186)
  line L2333 (31.5021, -2.1186) -> (31.4579, -2.0943)
  line L2334 (31.4579, -2.0943) -> (31.404, -2.0778)
  line L2335 (31.404, -2.0778) -> (31.341, -2.0699)
  line L2336 (31.341, -2.0699) -> (31.2695, -2.0712)
  line L2337 (31.2695, -2.0712) -> (31.1903, -2.0825)
  line L2338 (31.1903, -2.0825) -> (31.104, -2.1043)
  line L2339 (31.104, -2.1043) -> (31.0114, -2.1374)
  line L2340 (31.0114, -2.1374) -> (30.9133, -2.1822)
  line L2341 (30.9133, -2.1822) -> (30.8106, -2.2393)
  line L2342 (30.8106, -2.2393) -> (30.762, -2.2546)
  line L2343 (30.762, -2.2546) -> (30.6724, -2.2738)
  line L2344 (30.6724, -2.2738) -> (30.5422, -2.2905)
  line L2345 (30.5422, -2.2905) -> (30.4624, -2.2959)
  line L2346 (30.4624, -2.2959) -> (30.3717, -2.2981)
  line L2347 (30.3717, -2.2981) -> (30.2725, -2.2965)
  line L2348 (30.2725, -2.2965) -> (30.1616, -2.2899)
  line L2349 (30.1616, -2.2899) -> (30.0431, -2.278)
  line L2350 (30.0431, -2.278) -> (29.9141, -2.2595)
  line L2351 (29.9141, -2.2595) -> (29.7768, -2.2339)
  line L2352 (29.7768, -2.2339) -> (29.6305, -2.2002)
  line L2353 (29.6305, -2.2002) -> (29.4762, -2.1578)
  line L2354 (29.4762, -2.1578) -> (29.3255, -2.1096)
  arc A76 (29.1649, -1.5103) -> (29.3255, -2.1096) centre (36, 0) ccw
  line L2355 (29.1649, -1.5103) -> (29.2713, -1.3932)
  line L2356 (29.2713, -1.3932) -> (29.3837, -1.2793)
  line L2357 (29.3837, -1.2793) -> (29.4936, -1.177)
  line L2358 (29.4936, -1.177) -> (29.5997, -1.0861)
  line L2359 (29.5997, -1.0861) -> (29.7022, -1.0056)
  line L2360 (29.7022, -1.0056) -> (29.7988, -0.9361)
  line L2361 (29.7988, -0.9361) -> (29.8916, -0.875)
  line L2362 (29.8916, -0.875) -> (29.9767, -0.8239)
  line L2363 (29.9767, -0.8239) -> (30.0563, -0.7805)
  line L2364 (30.0563, -0.7805) -> (30.1282, -0.7452)
  line L2365 (30.1282, -0.7452) -> (30.2493, -0.6947)
  line L2366 (30.2493, -0.6947) -> (30.3365, -0.6665)
  line L2367 (30.3365, -0.6665) -> (30.3862, -0.6555)
  line L2368 (30.3862, -0.6555) -> (30.5037, -0.6535)
  line L2369 (30.5037, -0.6535) -> (30.611, -0.6433)
  line L2370 (30.611, -0.6433) -> (30.7078, -0.6256)
  line L2371 (30.7078, -0.6256) -> (30.7934, -0.6014)
  line L2372 (30.7934, -0.6014) -> (30.8677, -0.5716)
  line L2373 (30.8677, -0.5716) -> (30.9302, -0.537)
  line L2374 (30.9302, -0.537) -> (30.9808, -0.4986)
  line L2375 (30.9808, -0.4986) -> (31.0192, -0.4573)
  line L2376 (31.0192, -0.4573) -> (31.0454, -0.4142)
  line L2377 (31.0454, -0.4142) -> (31.0592, -0.3701)
  line L2378 (31.0592, -0.3701) -> (31.0614, -0.337)
  line L2379 (31.0614, -0.337) -> (31.0529, -0.1693)
  line L2380 (31.0529, -0.1693) -> (31.05, 0)
  line L2381 (31.05, 0) -> (31.0529, 0.1693)
  line L2382 (31.0529, 0.1693) -> (31.0614, 0.337)
  line L2383 (31.0614, 0.337) -> (31.0592, 0.3701)
  line L2384 (31.0592, 0.3701) -> (31.0454, 0.4142)
  line L2385 (31.0454, 0.4142) -> (31.0192, 0.4573)
  line L2386 (31.0192, 0.4573) -> (30.9808, 0.4986)
  line L2387 (30.9808, 0.4986) -> (30.9302, 0.537)
  line L2388 (30.9302, 0.537) -> (30.8677, 0.5716)
  line L2389 (30.8677, 0.5716) -> (30.7934, 0.6014)
  line L2390 (30.7934, 0.6014) -> (30.7078, 0.6256)
  line L2391 (30.7078, 0.6256) -> (30.611, 0.6433)
  line L2392 (30.611, 0.6433) -> (30.5037, 0.6535)
  line L2393 (30.5037, 0.6535) -> (30.3862, 0.6555)
  line L2394 (30.3862, 0.6555) -> (30.3365, 0.6665)
  line L2395 (30.3365, 0.6665) -> (30.2493, 0.6947)
  line L2396 (30.2493, 0.6947) -> (30.1282, 0.7452)
  line L2397 (30.1282, 0.7452) -> (30.0563, 0.7805)
  line L2398 (30.0563, 0.7805) -> (29.9767, 0.8239)
  line L2399 (29.9767, 0.8239) -> (29.8916, 0.875)
  line L2400 (29.8916, 0.875) -> (29.7988, 0.9361)
  line L2401 (29.7988, 0.9361) -> (29.7022, 1.0056)
  line L2402 (29.7022, 1.0056) -> (29.5997, 1.0861)
  line L2403 (29.5997, 1.0861) -> (29.4936, 1.177)
  line L2404 (29.4936, 1.177) -> (29.3837, 1.2793)
  line L2405 (29.3837, 1.2793) -> (29.2713, 1.3932)
  line L2406 (29.2713, 1.3932) -> (29.1649, 1.5103)
  arc A77 (29.3255, 2.1096) -> (29.1649, 1.5103) centre (36, 0) ccw
  line L2407 (29.3255, 2.1096) -> (29.4762, 2.1578)
  line L2408 (29.4762, 2.1578) -> (29.6305, 2.2002)
  line L2409 (29.6305, 2.2002) -> (29.7768, 2.2339)
  line L2410 (29.7768, 2.2339) -> (29.9141, 2.2595)
  line L2411 (29.9141, 2.2595) -> (30.0431, 2.278)
  line L2412 (30.0431, 2.278) -> (30.1616, 2.2899)
  line L2413 (30.1616, 2.2899) -> (30.2725, 2.2965)
  line L2414 (30.2725, 2.2965) -> (30.3717, 2.2981)
  line L2415 (30.3717, 2.2981) -> (30.4624, 2.2959)
  line L2416 (30.4624, 2.2959) -> (30.5422, 2.2905)
  line L2417 (30.5422, 2.2905) -> (30.6724, 2.2738)
  line L2418 (30.6724, 2.2738) -> (30.762, 2.2546)
  line L2419 (30.762, 2.2546) -> (30.8106, 2.2393)
  line L2420 (30.8106, 2.2393) -> (30.9133, 2.1822)
  line L2421 (30.9133, 2.1822) -> (31.0114, 2.1374)
  line L2422 (31.0114, 2.1374) -> (31.104, 2.1043)
  line L2423 (31.104, 2.1043) -> (31.1903, 2.0825)
  line L2424 (31.1903, 2.0825) -> (31.2695, 2.0712)
  line L2425 (31.2695, 2.0712) -> (31.341, 2.0699)
  line L2426 (31.341, 2.0699) -> (31.404, 2.0778)
  line L2427 (31.404, 2.0778) -> (31.4579, 2.0943)
  line L2428 (31.4579, 2.0943) -> (31.5021, 2.1186)
  line L2429 (31.5021, 2.1186) -> (31.5361, 2.1499)
  line L2430 (31.5361, 2.1499) -> (31.5546, 2.1774)
  line L2431 (31.5546, 2.1774) -> (31.631, 2.327)
  line L2432 (31.631, 2.327) -> (31.7132, 2.475)
  line L2433 (31.7132, 2.475) -> (31.8003, 2.6202)
  line L2434 (31.8003, 2.6202) -> (31.8916, 2.7611)
  line L2435 (31.8916, 2.7611) -> (31.9062, 2.7909)
  line L2436 (31.9062, 2.7909) -> (31.9163, 2.836)
  line L2437 (31.9163, 2.836) -> (31.9152, 2.8864)
  line L2438 (31.9152, 2.8864) -> (31.9025, 2.9414)
  line L2439 (31.9025, 2.9414) -> (31.8779, 2.9999)
  line L2440 (31.8779, 2.9999) -> (31.841, 3.0611)
  line L2441 (31.841, 3.0611) -> (31.7917, 3.1241)
  line L2442 (31.7917, 3.1241) -> (31.7296, 3.1879)
  line L2443 (31.7296, 3.1879) -> (31.6547, 3.2516)
  line L2444 (31.6547, 3.2516) -> (31.5668, 3.3141)
  line L2445 (31.5668, 3.3141) -> (31.466, 3.3746)
  line L2446 (31.466, 3.3746) -> (31.4285, 3.4089)
  line L2447 (31.4285, 3.4089) -> (31.3671, 3.477)
  line L2448 (31.3671, 3.477) -> (31.2875, 3.5813)
  line L2449 (31.2875, 3.5813) -> (31.2429, 3.6478)
  line L2450 (31.2429, 3.6478) -> (31.1956, 3.7252)
  line L2451 (31.1956, 3.7252) -> (31.1475, 3.8119)
  line L2452 (31.1475, 3.8119) -> (31.0977, 3.9112)
  line L2453 (31.0977, 3.9112) -> (31.0488, 4.0198)
  line L2454 (31.0488, 4.0198) -> (31.0003, 4.1408)
  line L2455 (31.0003, 4.1408) -> (30.9538, 4.2725)
  line L2456 (30.9538, 4.2725) -> (30.9098, 4.4161)
  line L2457 (30.9098, 4.4161) -> (30.8694, 4.5708)
  line L2458 (30.8694, 4.5708) -> (30.8358, 4.7255)
  arc A78 (31.2745, 5.1642) -> (30.8358, 4.7255) centre (36, 0) ccw
  line L2459 (31.2745, 5.1642) -> (31.4292, 5.1306)
  line L2460 (31.4292, 5.1306) -> (31.5839, 5.0902)
  line L2461 (31.5839, 5.0902) -> (31.7275, 5.0462)
  line L2462 (31.7275, 5.0462) -> (31.8592, 4.9997)
  line L2463 (31.8592, 4.9997) -> (31.9802, 4.9512)
  line L2464 (31.9802, 4.9512) -> (32.0888, 4.9023)
  line L2465 (32.0888, 4.9023) -> (32.1881, 4.8525)
  line L2466 (32.1881, 4.8525) -> (32.2748, 4.8044)
  line L2467 (32.2748, 4.8044) -> (32.3522, 4.7571)
  line L2468 (32.3522, 4.7571) -> (32.4187, 4.7125)
  line L2469 (32.4187, 4.7125) -> (32.523, 4.6329)
  line L2470 (32.523, 4.6329) -> (32.5911, 4.5715)
  line L2471 (32.5911, 4.5715) -> (32.6254, 4.534)
  line L2472 (32.6254, 4.534) -> (32.6859, 4.4332)
  line L2473 (32.6859, 4.4332) -> (32.7484, 4.3453)
  line L2474 (32.7484, 4.3453) -> (32.8121, 4.2704)
  line L2475 (32.8121, 4.2704) -> (32.8759, 4.2083)
  line L2476 (32.8759, 4.2083) -> (32.9389, 4.159)
  line L2477 (32.9389, 4.159) -> (33.0001, 4.1221)
  line L2478 (33.0001, 4.1221) -> (33.0586, 4.0975)
  line L2479 (33.0586, 4.0975) -> (33.1136, 4.0848)
  line L2480 (33.1136, 4.0848) -> (33.164, 4.0837)
  line L2481 (33.164, 4.0837) -> (33.2091, 4.0938)
  line L2482 (33.2091, 4.0938) -> (33.2389, 4.1084)
  line L2483 (33.2389, 4.1084) -> (33.3798, 4.1997)
  line L2484 (33.3798, 4.1997) -> (33.525, 4.2868)
  line L2485 (33.525, 4.2868) -> (33.673, 4.369)
  line L2486 (33.673, 4.369) -> (33.8226, 4.4454)
  line L2487 (33.8226, 4.4454) -> (33.8501, 4.4639)
  line L2488 (33.8501, 4.4639) -> (33.8814, 4.4979)
  line L2489 (33.8814, 4.4979) -> (33.9057, 4.5421)
  line L2490 (33.9057, 4.5421) -> (33.9222, 4.596)
  line L2491 (33.9222, 4.596) -> (33.9301, 4.659)
  line L2492 (33.9301, 4.659) -> (33.9288, 4.7305)
  line L2493 (33.9288, 4.7305) -> (33.9175, 4.8097)
  line L2494 (33.9175, 4.8097) -> (33.8957, 4.896)
  line L2495 (33.8957, 4.896) -> (33.8626, 4.9886)
  line L2496 (33.8626, 4.9886) -> (33.8178, 5.0867)
  line L2497 (33.8178, 5.0867) -> (33.7607, 5.1894)
  line L2498 (33.7607, 5.1894) -> (33.7454, 5.238)
  line L2499 (33.7454, 5.238) -> (33.7262, 5.3276)
  line L2500 (33.7262, 5.3276) -> (33.7095, 5.4578)
  line L2501 (33.7095, 5.4578) -> (33.7041, 5.5376)
  line L2502 (33.7041, 5.5376) -> (33.7019, 5.6283)
  line L2503 (33.7019, 5.6283) -> (33.7035, 5.7275)
  line L2504 (33.7035, 5.7275) -> (33.7101, 5.8384)
  line L2505 (33.7101, 5.8384) -> (33.722, 5.9569)
  line L2506 (33.722, 5.9569) -> (33.7405, 6.0859)
  line L2507 (33.7405, 6.0859) -> (33.7661, 6.2232)
  line L2508 (33.7661, 6.2232) -> (33.7998, 6.3695)
  line L2509 (33.7998, 6.3695) -> (33.8422, 6.5238)
  line L2510 (33.8422, 6.5238) -> (33.8904, 6.6745)
  arc A79 (34.4897, 6.8351) -> (33.8904, 6.6745) centre (36, 0) ccw
  line L2511 (34.4897, 6.8351) -> (34.6069, 6.7287)
  line L2512 (34.6069, 6.7287) -> (34.7207, 6.6163)
  line L2513 (34.7207, 6.6163) -> (34.823, 6.5064)
  line L2514 (34.823, 6.5064) -> (34.9138, 6.4003)
  line L2515 (34.9138, 6.4003) -> (34.9944, 6.2978)
  line L2516 (34.9944, 6.2978) -> (35.0639, 6.2012)
  line L2517 (35.0639, 6.2012) -> (35.125, 6.1084)
  line L2518 (35.125, 6.1084) -> (35.1761, 6.0233)
  line L2519 (35.1761, 6.0233) -> (35.2195, 5.9436)
  line L2520 (35.2195, 5.9436) -> (35.2548, 5.8718)
  line L2521 (35.2548, 5.8718) -> (35.3053, 5.7507)
  line L2522 (35.3053, 5.7507) -> (35.3335, 5.6635)
  line L2523 (35.3335, 5.6635) -> (35.3445, 5.6138)
  line L2524 (35.3445, 5.6138) -> (35.3465, 5.4963)
  line L2525 (35.3465, 5.4963) -> (35.3567, 5.389)
  line L2526 (35.3567, 5.389) -> (35.3744, 5.2923)
  line L2527 (35.3744, 5.2923) -> (35.3986, 5.2066)
  line L2528 (35.3986, 5.2066) -> (35.4284, 5.1323)
  line L2529 (35.4284, 5.1323) -> (35.463, 5.0698)
  line L2530 (35.463, 5.0698) -> (35.5014, 5.0192)
  line L2531 (35.5014, 5.0192) -> (35.5427, 4.9808)
  line L2532 (35.5427, 4.9808) -> (35.5858, 4.9546)
  line L2533 (35.5858, 4.9546) -> (35.6299, 4.9408)
  line L2534 (35.6299, 4.9408) -> (35.663, 4.9386)
  line L2535 (35.663, 4.9386) -> (35.8307, 4.9471)
  line L2536 (35.8307, 4.9471) -> (36, 4.95)
  line L2537 (36, 4.95) -> (36.1693, 4.9471)
  line L2538 (36.1693, 4.9471) -> (36.337, 4.9386)
  line L2539 (36.337, 4.9386) -> (36.3701, 4.9408)
  line L2540 (36.3701, 4.9408) -> (36.4142, 4.9546)
  line L2541 (36.4142, 4.9546) -> (36.4573, 4.9808)
  line L2542 (36.4573, 4.9808) -> (36.4986, 5.0192)
  line L2543 (36.4986, 5.0192) -> (36.537, 5.0698)
  line L2544 (36.537, 5.0698) -> (36.5716, 5.1323)
  line L2545 (36.5716, 5.1323) -> (36.6014, 5.2066)
  line L2546 (36.6014, 5.2066) -> (36.6256, 5.2923)
  line L2547 (36.6256, 5.2923) -> (36.6433, 5.389)
  line L2548 (36.6433, 5.389) -> (36.6535, 5.4963)
  line L2549 (36.6535, 5.4963) -> (36.6555, 5.6138)
  line L2550 (36.6555, 5.6138) -> (36.6665, 5.6635)
  line L2551 (36.6665, 5.6635) -> (36.6947, 5.7507)
  line L2552 (36.6947, 5.7507) -> (36.7452, 5.8718)
  line L2553 (36.7452, 5.8718) -> (36.7805, 5.9436)
  line L2554 (36.7805, 5.9436) -> (36.8239, 6.0233)
  line L2555 (36.8239, 6.0233) -> (36.875, 6.1084)
  line L2556 (36.875, 6.1084) -> (36.9361, 6.2012)
  line L2557 (36.9361, 6.2012) -> (37.0056, 6.2978)
  line L2558 (37.0056, 6.2978) -> (37.0862, 6.4003)
  line L2559 (37.0862, 6.4003) -> (37.177, 6.5064)
  line L2560 (37.177, 6.5064) -> (37.2793, 6.6163)
  line L2561 (37.2793, 6.6163) -> (37.3931, 6.7287)
  line L2562 (37.3931, 6.7287) -> (37.5103, 6.8351)
  arc A80 (38.1096, 6.6745) -> (37.5103, 6.8351) centre (36, 0) ccw
  line L2563 (38.1096, 6.6745) -> (38.1578, 6.5238)
  line L2564 (38.1578, 6.5238) -> (38.2002, 6.3695)
  line L2565 (38.2002, 6.3695) -> (38.2339, 6.2232)
  line L2566 (38.2339, 6.2232) -> (38.2595, 6.0859)
  line L2567 (38.2595, 6.0859) -> (38.278, 5.9569)
  line L2568 (38.278, 5.9569) -> (38.2899, 5.8384)
  line L2569 (38.2899, 5.8384) -> (38.2965, 5.7275)
  line L2570 (38.2965, 5.7275) -> (38.2981, 5.6283)
  line L2571 (38.2981, 5.6283) -> (38.2959, 5.5376)
  line L2572 (38.2959, 5.5376) -> (38.2905, 5.4578)
  line L2573 (38.2905, 5.4578) -> (38.2738, 5.3276)
  line L2574 (38.2738, 5.3276) -> (38.2546, 5.238)
  line L2575 (38.2546, 5.238) -> (38.2393, 5.1894)
  line L2576 (38.2393, 5.1894) -> (38.1822, 5.0867)
  line L2577 (38.1822, 5.0867) -> (38.1374, 4.9886)
  line L2578 (38.1374, 4.9886) -> (38.1043, 4.896)
  line L2579 (38.1043, 4.896) -> (38.0825, 4.8097)
  line L2580 (38.0825, 4.8097) -> (38.0712, 4.7305)
  line L2581 (38.0712, 4.7305) -> (38.0699, 4.659)
  line L2582 (38.0699, 4.659) -> (38.0778, 4.596)
  line L2583 (38.0778, 4.596) -> (38.0943, 4.5421)
  line L2584 (38.0943, 4.5421) -> (38.1186, 4.4979)
  line L2585 (38.1186, 4.4979) -> (38.1499, 4.4639)
  line L2586 (38.1499, 4.4639) -> (38.1774, 4.4454)
  line L2587 (38.1774, 4.4454) -> (38.327, 4.369)
  line L2588 (38.327, 4.369) -> (38.475, 4.2868)
  line L2589 (38.475, 4.2868) -> (38.6202, 4.1997)
  line L2590 (38.6202, 4.1997) -> (38.7611, 4.1084)
  line L2591 (38.7611, 4.1084) -> (38.7909, 4.0938)
  line L2592 (38.7909, 4.0938) -> (38.836, 4.0837)
  line L2593 (38.836, 4.0837) -> (38.8864, 4.0848)
  line L2594 (38.8864, 4.0848) -> (38.9414, 4.0975)
  line L2595 (38.9414, 4.0975) -> (38.9999, 4.1221)
  line L2596 (38.9999, 4.1221) -> (39.0611, 4.159)
  line L2597 (39.0611, 4.159) -> (39.1241, 4.2083)
  line L2598 (39.1241, 4.2083) -> (39.1879, 4.2704)
  line L2599 (39.1879, 4.2704) -> (39.2516, 4.3453)
  line L2600 (39.2516, 4.3453) -> (39.3141, 4.4332)
  line L2601 (39.3141, 4.4332) -> (39.3746, 4.534)
  line L2602 (39.3746, 4.534) -> (39.4089, 4.5715)
  line L2603 (39.4089, 4.5715) -> (39.477, 4.6329)
  line L2604 (39.477, 4.6329) -> (39.5813, 4.7125)
  line L2605 (39.5813, 4.7125) -> (39.6478, 4.7571)
  line L2606 (39.6478, 4.7571) -> (39.7252, 4.8044)
  line L2607 (39.7252, 4.8044) -> (39.8119, 4.8525)
  line L2608 (39.8119, 4.8525) -> (39.9112, 4.9023)
  line L2609 (39.9112, 4.9023) -> (40.0198, 4.9512)
  line L2610 (40.0198, 4.9512) -> (40.1408, 4.9997)
  line L2611 (40.1408, 4.9997) -> (40.2725, 5.0462)
  line L2612 (40.2725, 5.0462) -> (40.4161, 5.0902)
  line L2613 (40.4161, 5.0902) -> (40.5708, 5.1306)
  line L2614 (40.5708, 5.1306) -> (40.7255, 5.1642)
  arc A81 (41.1642, 4.7255) -> (40.7255, 5.1642) centre (36, 0) ccw
  line L2615 (41.1642, 4.7255) -> (41.1306, 4.5708)
  line L2616 (41.1306, 4.5708) -> (41.0902, 4.4161)
  line L2617 (41.0902, 4.4161) -> (41.0462, 4.2725)
  line L2618 (41.0462, 4.2725) -> (40.9997, 4.1408)
  line L2619 (40.9997, 4.1408) -> (40.9512, 4.0198)
  line L2620 (40.9512, 4.0198) -> (40.9023, 3.9112)
  line L2621 (40.9023, 3.9112) -> (40.8525, 3.8119)
  line L2622 (40.8525, 3.8119) -> (40.8044, 3.7252)
  line L2623 (40.8044, 3.7252) -> (40.7571, 3.6478)
  line L2624 (40.7571, 3.6478) -> (40.7125, 3.5813)
  line L2625 (40.7125, 3.5813) -> (40.6329, 3.477)
  line L2626 (40.6329, 3.477) -> (40.5715, 3.4089)
  line L2627 (40.5715, 3.4089) -> (40.534, 3.3746)
  line L2628 (40.534, 3.3746) -> (40.4332, 3.3141)
  line L2629 (40.4332, 3.3141) -> (40.3453, 3.2516)
  line L2630 (40.3453, 3.2516) -> (40.2704, 3.1879)
  line L2631 (40.2704, 3.1879) -> (40.2083, 3.1241)
  line L2632 (40.2083, 3.1241) -> (40.159, 3.0611)
  line L2633 (40.159, 3.0611) -> (40.1221, 2.9999)
  line L2634 (40.1221, 2.9999) -> (40.0975, 2.9414)
  line L2635 (40.0975, 2.9414) -> (40.0848, 2.8864)
  line L2636 (40.0848, 2.8864) -> (40.0837, 2.836)
  line L2637 (40.0837, 2.836) -> (40.0938, 2.7909)
  line L2638 (40.0938, 2.7909) -> (40.1084, 2.7611)
  line L2639 (40.1084, 2.7611) -> (40.1997, 2.6202)
  line L2640 (40.1997, 2.6202) -> (40.2868, 2.475)
  line L2641 (40.2868, 2.475) -> (40.369, 2.327)
  line L2642 (40.369, 2.327) -> (40.4454, 2.1774)
  line L2643 (40.4454, 2.1774) -> (40.4639, 2.1499)
  line L2644 (40.4639, 2.1499) -> (40.4979, 2.1186)
  line L2645 (40.4979, 2.1186) -> (40.5421, 2.0943)
  line L2646 (40.5421, 2.0943) -> (40.596, 2.0778)
  line L2647 (40.596, 2.0778) -> (40.659, 2.0699)
  line L2648 (40.659, 2.0699) -> (40.7305, 2.0712)
  line L2649 (40.7305, 2.0712) -> (40.8097, 2.0825)
  line L2650 (40.8097, 2.0825) -> (40.896, 2.1043)
  line L2651 (40.896, 2.1043) -> (40.9886, 2.1374)
  line L2652 (40.9886, 2.1374) -> (41.0867, 2.1822)
  line L2653 (41.0867, 2.1822) -> (41.1894, 2.2393)
  line L2654 (41.1894, 2.2393) -> (41.238, 2.2546)
  line L2655 (41.238, 2.2546) -> (41.3276, 2.2738)
  line L2656 (41.3276, 2.2738) -> (41.4578, 2.2905)
  line L2657 (41.4578, 2.2905) -> (41.5376, 2.2959)
  line L2658 (41.5376, 2.2959) -> (41.6283, 2.2981)
  line L2659 (41.6283, 2.2981) -> (41.7275, 2.2965)
  line L2660 (41.7275, 2.2965) -> (41.8384, 2.2899)
  line L2661 (41.8384, 2.2899) -> (41.9569, 2.278)
  line L2662 (41.9569, 2.278) -> (42.0859, 2.2595)
  line L2663 (42.0859, 2.2595) -> (42.2232, 2.2339)
  line L2664 (42.2232, 2.2339) -> (42.3695, 2.2002)
  line L2665 (42.3695, 2.2002) -> (42.5238, 2.1578)
  line L2666 (42.5238, 2.1578) -> (42.6745, 2.1096)
  arc A82 (42.8351, 1.5103) -> (42.6745, 2.1096) centre (36, 0) ccw
  line L2667 (42.8351, 1.5103) -> (42.7287, 1.3932)
  line L2668 (42.7287, 1.3932) -> (42.6163, 1.2793)
  line L2669 (42.6163, 1.2793) -> (42.5064, 1.177)
  line L2670 (42.5064, 1.177) -> (42.4003, 1.0861)
  line L2671 (42.4003, 1.0861) -> (42.2978, 1.0056)
  line L2672 (42.2978, 1.0056) -> (42.2012, 0.9361)
  line L2673 (42.2012, 0.9361) -> (42.1084, 0.875)
  line L2674 (42.1084, 0.875) -> (42.0233, 0.8239)
  line L2675 (42.0233, 0.8239) -> (41.9437, 0.7805)
  line L2676 (41.9437, 0.7805) -> (41.8718, 0.7452)
  line L2677 (41.8718, 0.7452) -> (41.7507, 0.6947)
  line L2678 (41.7507, 0.6947) -> (41.6635, 0.6665)
  line L2679 (41.6635, 0.6665) -> (41.6138, 0.6555)
  line L2680 (41.6138, 0.6555) -> (41.4963, 0.6535)
  line L2681 (41.4963, 0.6535) -> (41.389, 0.6433)
  line L2682 (41.389, 0.6433) -> (41.2923, 0.6256)
  line L2683 (41.2923, 0.6256) -> (41.2066, 0.6014)
  line L2684 (41.2066, 0.6014) -> (41.1323, 0.5716)
  line L2685 (41.1323, 0.5716) -> (41.0698, 0.537)
  line L2686 (41.0698, 0.537) -> (41.0192, 0.4986)